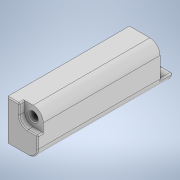
# Autodesk Inventor part: Corner-001A
Saved by Autodesk Inventor 2022 (Build 260153000, 153)
## iProperties
Created: 2024-01-30
Part Number: Corner-001A
Material: Generic
Document SubType Name: Modeling
Designer: Paul
Density: 1 g/cm^3
Appearance: Default
Author: Paul
Autodesk Inventor part; units mm, degrees
ref_plane "YZ Plane" through (0, 0, 0) normal (1, 0, 0) x (0, 1, 0)
ref_plane "XZ Plane" through (0, 0, 0) normal (0, 1, 0) x (-1, 0, 0)
ref_plane "XY Plane" through (0, 0, 0) normal (0, 0, 1) x (1, 0, 0)
sketch "Sketch1" plane through (0, 0, 0) normal (0, 0, 1) x (1, 0, 0)
  line L0 (0, 0) -> (25.4, 0)
  line L1 (25.4, 0) -> (25.4, 25.4)
  line L2 (25.4, 25.4) -> (0, 25.4)
  line L3 (0, 25.4) -> (0, 0)
  dimension "d0" = 25.4
  dimension "d1" = 25.4
  constraints: 8 end point, 2 parallel, 1 horizontal, 1 perpendicular
  measures "d0" distance of L1.end L2.end
  measures "d1" distance of L0.end L1.end
extrude "Extrusion1" add sketch "Sketch1" along normal blind 84.138
sketch "Sketch2" plane through (0, 0, 84.138) normal (0, 0, 1) x (1, 0, 0)
  line L0 (25.4, 25.4) -> (0, 25.4) projected
  line L1 (25.4, 25.4) -> (13.779, 25.4)
  line L2 (13.779, 25.4) -> (13.779, 13.779)
  line L3 (13.779, 13.779) -> (25.4, 13.779)
  line L4 (25.4, 13.779) -> (25.4, 25.4)
  point P0 (0, 0)
  dimension "d4" = 11.621
  dimension "d5" = 11.621
  constraints: 8 end point, 2 parallel, 1 horizontal, 1 perpendicular
  measures "d4" distance between parallel lines of L4 L2
  measures "d5" distance between parallel lines of L0 L3
extrude "Extrusion2" cut sketch "Sketch2" against normal blind 3.429
sketch "Sketch3" plane through (0, 0, 0) normal (0, 0, -1) x (-1, 0, 0)
  line L0 (-25.4, 25.4) -> (-25.4, 13.779) projected
  line L1 (-25.4, 25.4) -> (-5.842, 25.4)
  line L2 (-5.842, 25.4) -> (-5.842, 5.842)
  line L3 (-5.842, 5.842) -> (-25.4, 5.842)
  line L4 (-25.4, 5.842) -> (-25.4, 25.4)
  point P0 (0, 0)
  dimension "d8" = 19.558
  dimension "d9" = 19.558
  constraints: 8 end point, 2 parallel, 1 horizontal, 1 perpendicular
  measures "d8" distance between parallel lines of L0 L2
  measures "d9" distance between parallel lines of L1 L3
extrude "Extrusion3" cut sketch "Sketch3" against normal blind 7.938
sketch "Sketch4" plane through (0, 0, 7.938) normal (0, 0, -1) x (-1, 0, 0)
  line L0 (-25.4, 25.4) -> (-5.842, 25.4) projected
  line L1 (-25.4, 5.842) -> (-25.4, 25.4) projected
  point P0 (0, 0)
  point P1 (-19.05, 19.05)
  dimension "d12" = 6.35
  dimension "d13" = 6.35
  measures "d12" distance from line of point (-19.05, 19.05) L0
  measures "d13" distance from line of point (-19.05, 19.05) L1
hole "Hole1" at (19.05, 19.05, 7.938) direction (0, 0, 1) diameter 5.334 end through all clearance for "Flat Head Machine Screw (82)" size "#10" standard "Ansi Unified Screw Threads"
fillet "Fillet1" radius 6.35 4 edges at (0, 25.4, 42.069) (25.4, 25.4, 44.3235) (0, 0, 42.069) (25.4, 0, 42.069)
fillet "Fillet2" radius 0.794 4 edges at (25.3796, 5.842, 3.969) (5.842, 25.3796, 3.969) (25.4, 13.779, 82.4235) (13.779, 25.4, 82.4235)
fillet "Fillet3" radius 5.271 1 edges at (13.779, 13.779, 82.4235)
fillet "Fillet4" radius 13.208 1 edges at (5.842, 5.842, 3.969)
chamfer "Chamfer1" distance 0.6 angle 45 24 edges at (19.05, 16.383, 7.938) (9.7105, 9.7105, 0) (5.842, 21.7506, 0) (5.5393, 25.0751, 0) (1.3614, 22.9789, 0) (0, 12.7, 0) (1.8599, 1.8599, 0) (12.7, 0, 0) (22.9789, 1.3614, 0) (25.0751, 5.5393, 0) (21.7506, 5.842, 0) (19.05, 16.383, 80.709) (21.828, 13.779, 84.138) (15.3228, 15.3228, 84.138) (13.779, 21.828, 84.138) (13.5464, 25.1674, 84.138) (9.6675, 25.4, 84.138) (1.8599, 23.5401, 84.138) (0, 12.7, 84.138) (1.8599, 1.8599, 84.138) (12.7, 0, 84.138) (23.5401, 1.8599, 84.138) (25.4, 9.6675, 84.138) (25.1674, 13.5464, 84.138)
sketch "Sketch5" plane through (0, 0, 84.138) normal (0, 0, 1) x (1, 0, 0)
  line L0 (0, 0) -> (6.35, 0)
  line L1 (6.35, 0) -> (6.35, 25.4)
  line L2 (6.35, 25.4) -> (0, 25.4)
  line L3 (0, 25.4) -> (0, 0)
  dimension "d28" = 25.4
  dimension "d29" = 6.35
  constraints: 8 end point, 2 parallel, 1 horizontal, 1 perpendicular
  measures "d28" distance of L0.end L1.end
  measures "d29" distance of L1.end L2.end
extrude "Extrusion4" cut sketch "Sketch5" against normal through all
fillet "Fillet5" radius 0.794 1 edges at (6.35, 15.4222, 4.269)
chamfer "Chamfer2" distance 0.6 angle 45 3 edges at (6.35, 12.7, 84.138) (6.35, 6.1405, 0) (6.5098, 12.1586, 0)
equation "\"d5\" = d4"
equation "\"d9\" = d8"
equation "\"d13\" = d12"
body "Solid1"
